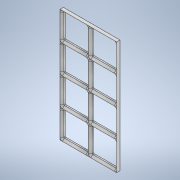
# Autodesk Inventor part: Single_frame
Saved by Autodesk Inventor 2021 (Build 250183000, 183)
## iProperties
Created: 2022-04-21
Part Number: Single_frame
Material: Generic
Document SubType Name: Modeling
Designer: Brice
Density: 1 g/cm^3
Appearance: Default
Author: Brice
Autodesk Inventor part; units mm, degrees
ref_plane "YZ Plane" through (0, 0, 0) normal (1, 0, 0) x (0, 1, 0)
ref_plane "XZ Plane" through (0, 0, 0) normal (0, 1, 0) x (-1, 0, 0)
ref_plane "XY Plane" through (0, 0, 0) normal (0, 0, 1) x (1, 0, 0)
sketch "Sketch1" plane through (0, 0, 0) normal (0, 0, 1) x (1, 0, 0)
  line L0 (21, -21) -> (63, -21)
  line L1 (63, -21) -> (63, -63)
  line L2 (63, -63) -> (21, -63)
  line L3 (21, -63) -> (21, -21)
  point P0 (0, 0)
  dimension "d7" = 42
  dimension "d8" = 42
  constraints: 8 end point, 2 parallel, 1 horizontal, 1 perpendicular
  measures "d7" distance of L2.end L0.start
  measures "d8" distance of L1.end L2.end
extrude "Extrusion1" add sketch "Sketch1" against normal blind 5
sketch "Sketch2" plane through (0, 0, -5) normal (0, 0, -1) x (-1, 0, 0)
  line L0 (-63, -63) -> (-21, -63) construction
  line L1 (-21, -21) -> (-63, -21) construction
  line L2 (-21, -63) -> (-63, -21) construction
  line L3 (-63, -63) -> (-21, -21) construction
  line L4 (-59.354, -23.846) -> (-24.646, -23.846)
  line L5 (-23.846, -24.646) -> (-23.846, -59.354)
  line L6 (-24.646, -60.154) -> (-59.354, -60.154)
  line L7 (-60.154, -59.354) -> (-60.154, -24.646)
  line L8 (-60.154, -23.846) -> (-23.846, -60.154) construction
  line L9 (-23.846, -23.846) -> (-60.154, -60.154) construction
  line L10 (-63, -21) -> (-63, -63) projected
  arc A0 (-59.354, -23.846) -> (-60.154, -24.646) centre (-59.354, -24.646) ccw
  arc A1 (-23.846, -24.646) -> (-24.646, -23.846) centre (-24.646, -24.646) ccw
  arc A2 (-24.646, -60.154) -> (-23.846, -59.354) centre (-24.646, -59.354) ccw
  arc A3 (-60.154, -59.354) -> (-59.354, -60.154) centre (-59.354, -59.354) ccw
  point P0 (0, 0)
  point P1 (-42, -42)
  dimension "d9" = 2.846
  dimension "d10" = 1.6
  dimension "d11" = 1.6
  dimension "d12" = 1.6
  dimension "d13" = 1.6
  constraints: 16 end point, 8 point on circle, 8 tangent, 5 point on line, 4 centre point, 3 midpoint, 2 parallel, 1 horizontal, 1 perpendicular
  measures "d9" distance between parallel lines of L7 L10
  measures "d10" diameter of A0
  measures "d11" diameter of A1
  measures "d12" diameter of A2
  measures "d13" diameter of A3
extrude "Extrusion2" cut sketch "Sketch2" against normal through all
chamfer "Chamfer2" distance 2.846 angle 45 8 edges at (42, -23.846, 0) (59.9197, -24.0803, 0) (60.154, -42, 0) (59.9197, -59.9197, 0) (42, -60.154, 0) (24.0803, -59.9197, 0) (23.846, -42, 0) (24.0803, -24.0803, 0)
pattern_linear "Rectangular Pattern1" count 4 spacing 42 along (0, -1, 0) count 2 spacing 42 along (1, 0, 0) of "Extrusion1", "Extrusion2", "Chamfer2"
equation "\"d7\" = CONST_Side_Length"
equation "\"d8\" = CONST_Side_Length"
equation "\"d9\" = CONST_Inset_Radius"
equation "\"d10\" = CONST_Curvature_Radius"
equation "\"d11\" = CONST_Curvature_Radius"
equation "\"d12\" = CONST_Curvature_Radius"
equation "\"d13\" = CONST_Curvature_Radius"
equation "\"d14\" = CONST_Inset_Radius"
equation "\"d19\" = CONST_Side_Length"
equation "\"d22\" = CONST_Side_Length"
equation "\"CONST_Side_Length\" = 42"
equation "\"CONST_Inset_Radius\" = 2.846"
equation "\"CONST_Curvature_Radius\" = 1.6"
body "Solid1"
